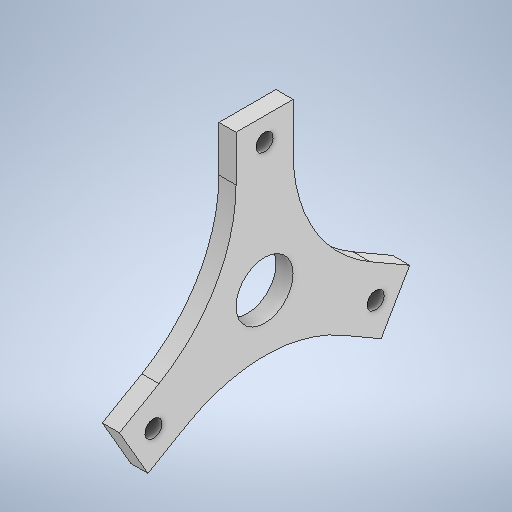
# Autodesk Inventor part: CAR_TRI_FRAME
Saved by Autodesk Inventor 2025.4 (Build 294407000, 407)
## iProperties
Created: 2026-07-11
Part Number: CAR_TRI_FRAME
Material: 常规
Document SubType Name: Sheet Metal
Designer: Admin
Density: 1 g/cm^3
Sheet Metal Rule: 默认_mm
Appearance: 默认
Mass: 2.44803 g
Surface Area: 23.2737 cm^2
Volume: 2.44803 cm^3
Author: Admin
Autodesk Inventor part; units mm, degrees
ref_plane "YZ Plane" through (0, 0, 0) normal (1, 0, 0) x (0, 1, 0)
ref_plane "XZ Plane" through (0, 0, 0) normal (0, 1, 0) x (-1, 0, 0)
ref_plane "XY Plane" through (0, 0, 0) normal (0, 0, 1) x (1, 0, 0)
sketch "草图1" plane through (0, 0, 0) normal (1, 0, 0) x (0, 1, 0)
  circle A0 centre (0, 0) radius 33.5
  circle A1 centre (33.5, 0) radius 5
  circle A2 centre (-16.75, 29.0119) radius 5
  circle A3 centre (-16.75, -29.0119) radius 5
  line L0 (33.5, 5) -> (18.5, 5)
  line L1 (18.5, 5) -> (18.5, -5)
  line L2 (18.5, -5) -> (33.5, -5)
  line L3 (33.5, -5) -> (33.5, 5)
  line L4 (-21.0801, 26.5119) -> (-13.5801, 13.5215)
  line L5 (-4.9199, 18.5215) -> (-12.4199, 31.5119)
  line L6 (-12.4199, -31.5119) -> (-4.9199, -18.5215)
  line L7 (-13.5801, -13.5215) -> (-21.0801, -26.5119)
  arc A4 (-4.9199, 18.5215) -> (18.5, 5) centre (18.5, 32.0429) ccw
  circle A5 centre (22.5, 0) radius 1.5
  line L8 (26.5, 5) -> (26.5, -5)
  arc A6 (-13.5801, -13.5215) -> (-13.5801, 13.5215) centre (-37, 0) ccw
  line L9 (-17.5801, 20.4497) -> (-8.9199, 25.4497)
  circle A7 centre (-11.25, 19.4856) radius 1.5
  arc A8 (18.5, -5) -> (-4.9199, -18.5215) centre (18.5, -32.0429) ccw
  line L10 (-8.9199, -25.4497) -> (-17.5801, -20.4497)
  circle A9 centre (-11.25, -19.4856) radius 1.5
  circle A10 centre (0, 0) radius 5
  point P0 (-4.9199, -18.5215)
  point P1 (18.5, -5)
  point P2 (-8.9199, 25.4497)
  point P3 (-13.5801, 13.5215)
  point P4 (-13.5801, -13.5215)
  point P5 (-17.5801, -20.4497)
  point P6 (-8.9199, -25.4497)
  dimension "d0" = 67
  dimension "d1" = 10
  dimension "d6" = 360
  dimension "d8" = 15
  dimension "d11" = 360
  dimension "d13" = 3
  dimension "d14" = 11
  dimension "d15" = 7
  dimension "d18" = 360
  dimension "d20" = 10
  constraints: 22 end point, 10 centre point, 8 point on circle, 3 horizontal alignment, 2 coincident, 2 parallel, 2 perpendicular, 2 point on line, 1 horizontal, 1 midpoint, 1 tangent, 1 vertical alignment, 56 other
  measures "d1" diameter of A1
  measures "d8" distance of L0.start L0.end
  measures "d13" diameter of A5
  measures "d14" distance of point (33.5, 0) A5.centre
  measures "d15" distance from line of A1.centre L8
  measures "d20" diameter of A10
extrude "拉伸1" add sketch "草图1" along normal blind 3 contours L8 L2 L1 L0 | L5 A4 L1 A8 L6 L10 L7 A6 L4 L9
equation "\"折弯半径\" = 厚度"
equation "\"折弯释压宽度\" = 厚度"
equation "\"折弯释压深度\" = 0.5 * 厚度"
equation "\"拐角释压尺寸\" = 4 * 厚度"
equation "\"最小余量\" = 2 * 厚度"
equation "\"过渡半径\" = 折弯半径"
equation "\"Jacobi半径尺寸\" = 折弯半径"
equation "\"间隙大小\" = 厚度"
equation "\"厚度\" = 0.5"
